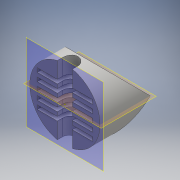
# Autodesk Inventor part: pipe_insert
Saved by Autodesk Inventor 2016 (Build 200138000, 138)
## iProperties
Created: 2016-04-05
Part Number: pipe_insert
Material: Generic
Document SubType Name: Modeling
Designer: 3DPrinterUser
Density: 1 g/cm^3
Appearance: Default
Author: 3DPrinterUser
Autodesk Inventor part; units mm, degrees
ref_plane "YZ Plane" through (0, 0, 0) normal (1, 0, 0) x (0, 1, 0)
sketch "Sketch1" plane through (0, 0, 0) normal (0, 1, 0) x (-1, 0, 0)
  circle A0 centre (0, 0) radius 35
  dimension "d0" = 70
  constraints: 1 centre point, 1 coincident
  measures "d0" diameter of A0
extrude "Extrusion1" add sketch "Sketch1" along normal blind 50
sketch "Sketch2" plane through (0, 0, 0) normal (1, 0, 0) x (0, 1, 0)
  point P0 (0, 0)
sketch "Sketch3" plane through (0, 0, 0) normal (0, 0, 1) x (1, 0, 0)
  line L0 (35, 50) -> (-35, 50) projected
  arc A0 (-35, 50) -> (35, 50) centre (0, 50) ccw
  point P0 (0, 0)
  dimension "d3" = 35
  constraints: 2 point on circle, 1 centre point
  measures "d3" radius of A0
extrude "Extrusion2" cut sketch "Sketch3" against normal blind 50 and the other way blind 50
sketch "Sketch4" plane through (0, 0, 0) normal (0, 0, 1) x (1, 0, 0)
  arc A0 (7.4545, 6.2837) -> (-7.5, 5.4589) centre (0, 5.4589) ccw
  line L0 (7.4545, 6.2837) -> (7.4545, 0)
  line L1 (-35, 0) -> (35, 0) projected
  line L2 (-7.5, 5.4589) -> (-7.5, 0)
  line L3 (-7.5, 0) -> (7.4545, 0)
  line L4 (7.4545, 0) -> (3.6133, 0)
  line L5 (3.6133, 0) -> (-3.6133, 0)
  line L6 (-3.6133, 0) -> (-7.5, 0)
  point P0 (0, 0)
  dimension "d8" = 15
  constraints: 12 end point, 4 point on line, 2 collinear, 2 point on circle, 1 centre point, 1 parallel, 1 tangent, 1 vertical
  measures "d8" diameter of A0
extrude "Extrusion3" cut sketch "Sketch4" along normal blind 50 and the other way blind 50
sketch "Sketch5" plane through (0, 0, 0) normal (0, 1, 0) x (-1, 0, 0)
  point P0 (0, 0)
sketch "Sketch6" plane through (0, 0, 0) normal (0, 1, 0) x (-1, 0, 0)
  line L0 (-27.5, -2) -> (27.5, -2)
  line L1 (27.5, -2) -> (27.5, 2)
  line L2 (27.5, 2) -> (-27.5, 2)
  line L3 (-27.5, 2) -> (-27.5, -2)
  line L4 (-27.5, -2) -> (27.5, 2) construction
  line L5 (27.5, -2) -> (-27.5, 2) construction
  line L6 (27.5, -6) -> (-27.5, -6)
  line L7 (-27.5, -6) -> (-27.5, -10)
  line L8 (-27.5, -10) -> (27.5, -10)
  line L9 (27.5, -10) -> (27.5, -6)
  line L10 (27.5, -14) -> (-27.5, -14)
  line L11 (-27.5, -14) -> (-27.5, -18)
  line L12 (-27.5, -18) -> (27.5, -18)
  line L13 (27.5, -18) -> (27.5, -14)
  line L14 (27.5, 10) -> (-27.5, 10)
  line L15 (-27.5, 10) -> (-27.5, 6)
  line L16 (-27.5, 6) -> (27.5, 6)
  line L17 (27.5, 6) -> (27.5, 10)
  line L18 (27.5, 2) -> (-27.5, 2)
  line L19 (-27.5, 2) -> (-27.5, -2)
  line L20 (-27.5, -2) -> (27.5, -2)
  line L21 (27.5, -2) -> (27.5, 2)
  line L22 (27.5, -6) -> (-27.5, -6)
  line L23 (-27.5, -6) -> (-27.5, -10)
  line L24 (-27.5, -10) -> (27.5, -10)
  line L25 (27.5, -10) -> (27.5, -6)
  line L26 (27.5, 18) -> (-27.5, 18)
  line L27 (-27.5, 18) -> (-27.5, 14)
  line L28 (-27.5, 14) -> (27.5, 14)
  line L29 (27.5, 14) -> (27.5, 18)
  line L30 (27.5, 10) -> (-27.5, 10)
  line L31 (-27.5, 10) -> (-27.5, 6)
  line L32 (-27.5, 6) -> (27.5, 6)
  line L33 (27.5, 6) -> (27.5, 10)
  line L34 (27.5, 2) -> (-27.5, 2)
  line L35 (-27.5, 2) -> (-27.5, -2)
  line L36 (-27.5, -2) -> (27.5, -2)
  line L37 (27.5, -2) -> (27.5, 2)
  point P0 (0, 0)
  dimension "d13" = 55
  dimension "d14" = 4
  dimension "d17" = 8
  dimension "d20" = 8
  constraints: 76 end point, 2 collinear, 2 midpoint, 2 parallel, 2 vertical, 1 horizontal, 1 perpendicular, 62 other
  measures "d13" distance of L2.end L1.end
  measures "d14" distance of L1.end L0.end
  measures "d17" distance of L1.end L6.start
  measures "d20" distance of L1.end L14.start
extrude "Extrusion4" cut sketch "Sketch6" along normal blind 50
body "Solid1"
